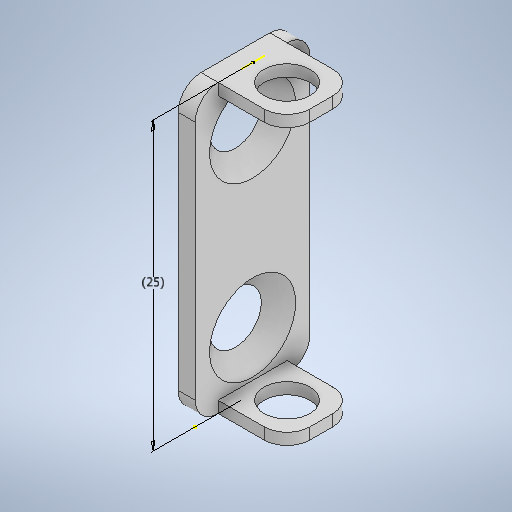
# Autodesk Inventor part: TRILHO LATERAL
Saved by Autodesk Inventor 2025.2 (Build 292293000, 293)
## iProperties
Created: 2025-05-13
Part Number: TRILHO LATERAL
Material: Genérico
Document SubType Name: Modeling
Designer: marce
Density: 1 g/cm^3
Appearance: Padrão
Author: marce
Autodesk Inventor part; units mm, degrees
ref_plane "YZ Plane" through (0, 0, 0) normal (1, 0, 0) x (0, 1, 0)
ref_plane "XZ Plane" through (0, 0, 0) normal (0, 1, 0) x (-1, 0, 0)
ref_plane "XY Plane" through (0, 0, 0) normal (0, 0, 1) x (1, 0, 0)
sketch "Esboço1" plane through (0, 0, 0) normal (1, 0, 0) x (0, 1, 0)
  line L0 (0, 0) -> (25, 0)
  line L1 (25, 0) -> (25, -10)
  line L2 (25, -10) -> (0, -10)
  line L3 (0, -10) -> (0, 0)
  point P0 (20.25, -5)
  point P1 (4.75, -5)
  dimension "d0" = 25
  dimension "d1" = 10
  constraints: 8 end point, 2 parallel, 1 horizontal, 1 perpendicular
  measures "d0" distance of L1.end L2.end
  measures "d1" distance of L0.end L1.end
extrude "Extrusão1" add sketch "Esboço1" along normal blind 1.5
fillet "Arredondamento1" radius 2 1 edges at (0.75, 25, 0)
fillet "Arredondamento2" radius 2 1 edges at (0.75, 25, -10)
fillet "Arredondamento3" radius 2 1 edges at (0.75, 0, 0)
fillet "Arredondamento4" radius 2 1 edges at (0.75, 0, -10)
sketch "Esboço2" plane through (1.5, 0, 0) normal (1, 0, 0) x (0, 0, -1)
  line L0 (8, 25) -> (2, 25) projected
  line L1 (5, 25) -> (5, 0)
  line L2 (2, 0) -> (8, 0) projected
  circle A0 centre (5, 5) radius 3.75
  circle A1 centre (5, 20.03) radius 3.75
  point P0 (0, 0)
  dimension "d12" = 4.97
  dimension "d13" = 5
  dimension "d15" = 7.5
  dimension "d16" = 7.5
  constraints: 3 midpoint, 2 centre point, 2 coincident, 2 end point, 2 point on line
  measures "d12" distance of point (5, 25) point (5, 20.03)
  measures "d13" distance from line of L2 point (5, 5)
  measures "d15" diameter of A0
  measures "d16" diameter of A1
hole "Furo1" at (1.5, 20.03, -5) at (1.5, 5, -5) direction (-1, 0, 0) diameter 4 depth 2 tip angle 118 countersink diameter 7.5 countersink angle 90
sketch "Esboço3" plane through (1.5, 0, 0) normal (1, 0, 0) x (0, 0, -1)
  arc A0 (8, 0) -> (10, 2) centre (8, 2) ccw projected
  line L0 (8, 0) -> (2, 0)
  line L1 (2, 0) -> (2, 1)
  line L2 (2, 1) -> (8, 1)
  line L3 (8, 1) -> (8, 0)
  point P0 (0, 0)
  dimension "d24" = 1
  dimension "d25" = 6
  constraints: 8 end point, 2 parallel, 1 horizontal, 1 perpendicular
  measures "d24" distance of L0.end L1.end
  measures "d25" distance of L1.end L2.end
extrude "Extrusão2" add sketch "Esboço3" along normal blind 6
fillet "Arredondamento5" radius 2 1 edges at (7.5, 0.5, -8)
fillet "Arredondamento6" radius 2 1 edges at (7.5, 0.5, -2)
pattern_linear "Padrão retangular1" count 2 spacing 24 along (0, 1, 0) of "Extrusão2"
fillet "Arredondamento7" radius 2 1 edges at (7.5, 24.5, -8)
fillet "Arredondamento8" radius 2 1 edges at (7.5, 24.5, -2)
sketch "Esboço4" plane through (0, 25, -2) normal (0, 1, 0) x (1, 0, 0)
  line L0 (1.5, 6) -> (5.5, 6) projected
  line L1 (1.5, 0) -> (5.5, 0) projected
  line L2 (7.5, 2) -> (7.5, 4) projected
  circle A0 centre (4.5, 3) radius 2
  point P0 (0, -2)
  dimension "d37" = 4
  constraints: 1 centre point
  measures "d37" diameter of A0
extrude "Extrusão3" cut sketch "Esboço4" against normal through all
sketch "Esboço5" plane through (1.5, 0, 0) normal (1, 0, 0) x (0, 0, -1)
  line L0 (6, 25) -> (4, 25) projected
  line L1 (4, 0) -> (6, 0) projected
  point P0 (0, 0)
  point P1 (5, 25)
  dimension "d40" = 25
  constraints: 1 midpoint
  measures "d40" distance from line of point (5, 25) L1
sketch "Esboço6" plane through (1.5, 0, 0) normal (1, 0, 0) x (0, 0, -1)
  point P0 (0, 0)
